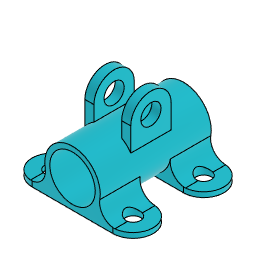
Exercise-14 v1 (Autodesk Fusion 360 design; units mm, degrees)
Autodesk Fusion 360 part; units mm, degrees
sketch "Sketch1" plane through (0, 0, 0) normal (0, 1, 0) x (1, 0, 0)
  circle A0 centre (0, 0) radius 22.5
  circle A1 centre (0, 0) radius 27.5
  line L0 (0, 0) -> (26.2268, -45.4262) construction
  line L1 (0, 0) -> (52.4536, 0) construction
  line L2 (22.75, -23.8157) -> (22.75, -58.8157)
  line L3 (22.75, -58.8157) -> (13.75, -58.8157)
  line L4 (13.75, -58.8157) -> (13.75, -23.8157)
  line L5 (22.75, -23.8157) -> (22.75, -15.4495)
  line L6 (0, 0) -> (0, -32.4408) construction
  line L7 (0, 0) -> (-26.2268, -45.4262) construction
  line L8 (-13.75, -58.8157) -> (-13.75, -23.8157)
  line L9 (-22.75, -23.8157) -> (-22.75, -58.8157)
  line L10 (-22.75, -23.8157) -> (-22.75, -15.4495)
  line L11 (-22.75, -58.8157) -> (-13.75, -58.8157)
  line L12 (60, 27.5) -> (-60, 27.5)
  line L13 (-60, 27.5) -> (-60, 22.5)
  line L14 (-60, 22.5) -> (60, 22.5)
  line L15 (60, 22.5) -> (60, 27.5)
  dimension "d1" = 45
  dimension "d2" = 55
  dimension "d3" = 60
  dimension "d4" = 9
  dimension "d5" = 35
  dimension "d6" = 120
  dimension "d7" = 5
  constraint coincident A0.centre A1.centre
  constraint concentric A0 A1
  constraint horizontal L1
  constraint vertical L2
  constraint horizontal L3
  constraint vertical L4
  constraint coincident A1 L4.end
  constraint coincident L0 L4.end
  constraint coincident A1 L5.end
  constraint perpendicular L1 L6
  constraint symmetric A0.centre L6 A1.centre
  constraint symmetric L0.end L6 L7.end
  constraint symmetric L4.end L6 L8.end
  constraint symmetric L2.start L6 L9.start
  constraint symmetric L2.end L6 L9.end
  constraint symmetric L3.end L6 L8.start
  constraint symmetric L5.end L6 L10.end
  constraint horizontal L12
  constraint perpendicular L12 L13
  constraint parallel L12 L14
  constraint parallel L13 L15
  measures "d1" diameter of A0
  measures "d2" diameter of A1
  measures "d3" angle of L0 L1
  measures "d4" distance of L4.end L2.start
  measures "d5" distance of L4.end L3.end
  measures "d6" distance of L13.end L14.end
  measures "d7" distance of L12.end L13.end
extrude "Extrude1" add sketch "Sketch1" along normal blind 110 contours A1 L14 | A1 L14
extrude "Extrude2" add sketch "Sketch1" along normal blind 40 from surface at 35 contours A1 L8 L9 L10 L11 | A1 L2 L3 L4 L5
extrude "Extrude3" add sketch "Sketch1" along normal blind 40 contours A1 L12 L13 L14 | A1 L12 L14 L15
fillet "Fillet1" radius 20 4 edges at (-18.25, 35, 58.8157) (18.25, 35, 58.8157) (-18.25, 75, 58.8157) (18.25, 75, 58.8157)
hole "Hole1" at (22.75, 55, 38.8157) direction (-1, 0, 0) diameter 20 end through all
fillet "Fillet2" radius 20 4 edges at (60, 0, -25) (60, 40, -25) (-60, 0, -25) (-60, 40, -25)
hole "Hole2" at (40, 20, -22.5) direction (0, 0, -1) diameter 15 end through all
hole "Hole3" at (-40, 20, -22.5) direction (0, 0, -1) diameter 15 end through all
fillet "Fillet3" radius 15 2 edges at (15.8114, 20, -22.5) (-15.8114, 20, -22.5)
pattern_linear "R-Pattern1" count 2 spacing 70 along (0, 1, 0) of "Extrude3", "Fillet2", "Hole2", "Hole3", "Fillet3"
